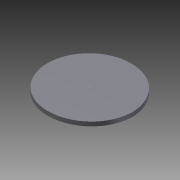
# Autodesk Inventor part: Disc Cam
Saved by Autodesk Inventor 2015 (Build 190159000, 159)
## iProperties
Created: 2015-04-14
Part Number: Disc Cam
Material: Stainless Steel, Austenitic
Document SubType Name: Modeling
Designer: WASHHSST
Manufacturer: Standard
Standards Organization: Custom
Density: 1 g/cm^3
Appearance: Steel
CustomPartVersion: 1
Author: WASHHSST
Autodesk Inventor part; units mm, degrees
ref_plane "YZ Plane" through (0, 0, 0) normal (1, 0, 0) x (0, 1, 0)
ref_plane "XZ Plane" through (0, 0, 0) normal (0, 1, 0) x (-1, 0, 0)
ref_plane "XY Plane" through (0, 0, 0) normal (0, 0, 1) x (1, 0, 0)
sketch "Main Sketch" plane through (0, 0, 0) normal (0, 0, 1) x (1, 0, 0)
  spline S0 degree 5 poles (0.6176, 127.0075) (3.7783, 127.045) (8.9531, 127.0041) (16.4373, 126.6845) (26.9375, 125.2035) (39.4178, 122.2697) (51.2949, 118.2021) (63.1244, 112.7723) (74.4186, 106.1348) (85.0034, 98.376) (94.7877, 89.5578) (103.6607, 79.7652) (111.518, 69.0982) (118.298, 57.6423) (123.8574, 45.5602) (128.2865, 32.8611) (131.1812, 19.9051) (133.321, 6.244) (132.8577, -6.71) (131.3997, -20.885) (128.1003, -34.3764) (123.3445, -47.78) (117.0161, -60.5385) (109.2718, -72.6091) (100.2043, -83.737) (89.972, -93.7983) (78.7323, -102.6552) (66.6673, -110.2177) (53.9523, -116.421) (40.7847, -121.2278) (27.3059, -124.6387) (13.7451, -126.6531) (0.0819, -127.3399) (-13.2121, -126.6673) (-26.4665, -124.5694) (-39.3421, -121.1189) (-51.7998, -116.3383) (-63.6733, -110.2874) (-74.8541, -103.0272) (-85.2127, -94.6386) (-94.6386, -85.2129) (-103.0272, -74.8537) (-110.2872, -63.6743) (-116.3388, -51.7974) (-121.1158, -39.3529) (-124.5658, -26.4773) (-126.6511, -13.3116) (-127.3487, 0) (-126.6511, 13.3116) (-124.5658, 26.4773) (-121.1158, 39.3529) (-116.3389, 51.7974) (-110.287, 63.6743) (-103.0277, 74.8538) (-94.6374, 85.2126) (-85.2155, 94.6393) (-74.8476, 103.0255) (-63.6884, 110.2912) (-51.7537, 116.335) (-39.8883, 120.9582) (-26.7368, 124.4185) (-16.5798, 126.2643) (-8.1331, 126.7958) (-2.6307, 126.9689) (0.6176, 127.0075) knots 0 0 0 0 0 0 0.019573 0.03264 0.048985 0.065356 0.081753 0.098176 0.114625 0.1311 0.147602 0.164129 0.180683 0.197264 0.213871 0.230462 0.24713 0.263884 0.280734 0.297684 0.314779 0.331924 0.349102 0.366296 0.383486 0.400652 0.417778 0.434848 0.451847 0.468767 0.485584 0.502314 0.518973 0.53558 0.552153 0.568725 0.585298 0.601871 0.618444 0.635017 0.65159 0.668163 0.684735 0.701308 0.717881 0.734454 0.751027 0.7676 0.784173 0.800745 0.817318 0.833891 0.850464 0.867037 0.88361 0.900183 0.916755 0.933328 0.949901 0.96655 0.979884 1 1 1 1 1 1
  point P0 (26.2495, 125.0364)
  point P1 (38.8454, 122.112)
  point P2 (51.1208, 117.9192)
  point P3 (62.948, 112.4926)
  point P4 (74.203, 105.8799)
  point P5 (84.7668, 98.1409)
  point P6 (94.5266, 89.3476)
  point P7 (103.3772, 79.5831)
  point P8 (111.2218, 68.9412)
  point P9 (117.9733, 57.5253)
  point P10 (123.5552, 45.4474)
  point P11 (127.9025, 32.8271)
  point P12 (130.9624, 19.7906)
  point P13 (132.6948, 6.4688)
  point P14 (132.61, -6.6688)
  point P15 (130.9907, -20.4975)
  point P16 (127.7802, -34.182)
  point P17 (122.9969, -47.5192)
  point P18 (116.6938, -60.3067)
  point P19 (108.958, -72.3512)
  point P20 (99.9077, -83.4757)
  point P21 (89.6877, -93.5259)
  point P22 (78.4631, -102.3757)
  point P23 (66.4119, -109.9295)
  point P24 (53.7176, -116.1234)
  point P25 (40.562, -120.9235)
  point P26 (27.119, -124.3231)
  point P27 (13.5497, -126.3377)
  point P28 (0, -127)
  point P29 (-13.2751, -126.3043)
  point P30 (-26.4048, -124.2247)
  point P31 (-39.2452, -120.7842)
  point P32 (-51.6556, -116.0203)
  point P33 (-63.5, -109.9852)
  point P34 (-74.6487, -102.7452)
  point P35 (-84.9796, -94.3794)
  point P36 (-94.3794, -84.9796)
  point P37 (-102.7452, -74.6487)
  point P38 (-109.9852, -63.5)
  point P39 (-116.0203, -51.6556)
  point P40 (-120.7842, -39.2452)
  point P41 (-124.2247, -26.4048)
  point P42 (-126.3043, -13.2751)
  point P43 (-127, 0)
  point P44 (-126.3043, 13.2751)
  point P45 (-124.2247, 26.4048)
  point P46 (-120.7842, 39.2452)
  point P47 (-116.0203, 51.6556)
  point P48 (-109.9852, 63.5)
  point P49 (-102.7452, 74.6487)
  point P50 (-94.3794, 84.9796)
  point P51 (-84.9796, 94.3794)
  point P52 (-74.6487, 102.7452)
  point P53 (-63.5, 109.9852)
  point P54 (-51.6556, 116.0203)
  point P55 (-39.2452, 120.7842)
  point P56 (-26.4048, 124.2247)
  point P57 (-13.2751, 126.3043)
  constraints: 60 other
extrude "Cam" add sketch "Main Sketch" along normal blind 12.7
body "Solid1"
